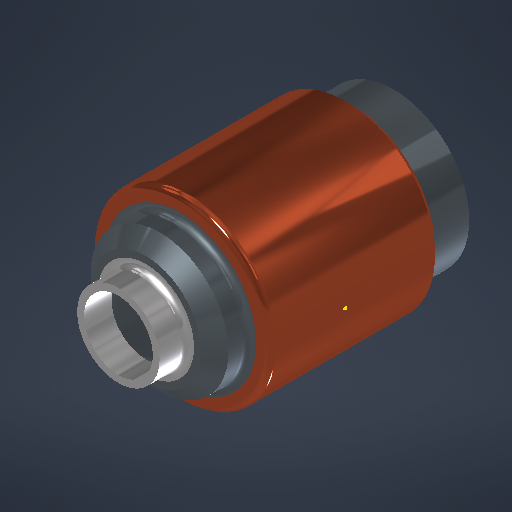
# Autodesk Inventor part: LOWER-NOZZLEv2
Saved by Autodesk Inventor 2025.3 (Build 293356030, 356C)
## iProperties
Created: 2025-08-29
Part Number: LOWER-NOZZLEv2
Material: PC/ABS Plastic
Document SubType Name: Modeling
Designer: lstk1ng
Density: 1.1 g/cm^3
Appearance: Smooth - White
Mass: 704.621 g
Surface Area: 1851.7 cm^2
Volume: 640.564 cm^3
Author: lstk1ng
Autodesk Inventor part; units mm, degrees
ref_plane "XZ Plane" through (0, 0, 0) normal (0, 1, 0) x (-1, 0, 0)
ref_plane "XY Plane" through (0, 0, 0) normal (0, 0, 1) x (1, 0, 0)
sketch "Sketch6" plane through (0, 0, 0) normal (0, 1, 0) x (-1, 0, 0)
  line L0 (0, -100) -> (0, 100)
  line L1 (50, -100) -> (50, -65)
  line L2 (60, -60) -> (60, 0.4584)
  line L3 (55, -65) -> (50, -65)
  line L4 (60, 50) -> (45, 50) construction
  line L5 (25, 80) -> (25, 100)
  line L6 (30, 100) -> (30, 85)
  line L7 (55, 55) -> (60, 55)
  line L8 (65, 50) -> (65, -65)
  line L9 (55, -100) -> (50, -100)
  line L10 (30, 100) -> (25, 100)
  line L11 (45, 50) -> (45, 50)
  line L12 (25, 80) -> (25, 80)
  line L13 (45, 50) -> (25, 80)
  arc A0 (65, 50) -> (60, 55) centre (60, 50) ccw
  arc A1 (50, 60) -> (55, 55) centre (55, 60) ccw
  line L14 (65, -65) -> (60, -70)
  line L15 (60, -60) -> (55, -65)
  line L16 (60, 45) -> (60, 45)
  line L17 (55, 50) -> (55, 50)
  line L18 (35, 80) -> (40, 80)
  line L19 (50, 70) -> (50, 60)
  line L20 (40, 80) -> (50, 70)
  line L21 (54.95, -100) -> (54.95, -70)
  line L22 (60, -70) -> (54.95, -70)
  arc A2 (30, 85) -> (35, 80) centre (35, 85) ccw
  arc A3 (60, 0.4584) -> (45, 50) centre (-29.3125, 0.4584) ccw
  point P0 (0, 0)
  point P1 (0, 0)
  point P2 (60, -65)
  point P3 (30, 80)
  point P4 (65, -70)
  point P5 (25, 50)
  point P6 (50, 80)
  dimension "d88" = 200
  dimension "d89" = 35
  dimension "d90" = 115
  dimension "d91" = 100
  dimension "d92" = 120
  dimension "d95" = 50
  dimension "d96" = 20
  dimension "d97" = 30
  dimension "d99" = 5
  dimension "d100" = 5
  dimension "d101" = 5
  dimension "d102" = 5
  dimension "d103" = 5
  dimension "d107" = 10
  dimension "d108" = 10
  dimension "d109" = 109.9
  dimension "d127" = 5
  constraints: 46 end point, 14 point on line, 8 point on circle, 7 tangent, 5 horizontal, 5 vertical, 4 centre point, 4 perpendicular, 1 coincident, 1 midpoint
  measures "d88" distance of L0.start L0.end
  measures "d89" distance of L1.start L1.end
  measures "d90" distance of L4.start point (60, -65)
  measures "d91" diameter of L1 L0
  measures "d92" diameter of L2 L0
  measures "d95" diameter of L5 L0
  measures "d96" distance of L11.end point (25, 50)
  measures "d97" distance of L12.start point (25, 50)
  measures "d99" distance of L8.end point (65, -70)
  measures "d100" distance of L14.end point (65, -70)
  measures "d101" distance of L2.start point (60, -65)
  measures "d102" distance of L3.start point (60, -65)
  measures "d103" distance of L16.end A0.centre
  measures "d107" distance of L18.end point (50, 80)
  measures "d108" distance of L19.start point (50, 80)
  measures "d109" diameter of L21 L0
  measures "d127" radius of A2
revolve "Revolution5" add sketch "Sketch6" angle 360 about axis through (0, 0, -100) along (0, 0, 1)
ref_plane "Work Plane2" through (65, 0, -7.5) normal (1, 0, 0) x (0, 1, 0)
sketch "Sketch17" plane through (65, 0, -7.5) normal (1, 0, 0) x (0, 1, 0)
  point P0 (0, 7.5)
ref_plane "Work Plane5" through (57.6628, -30, -7.5) normal (0, 0, -1) x (-1, 0, 0)
sketch "Sketch19" plane through (57.6628, -30, -7.5) normal (0, 0, -1) x (-1, 0, 0)
  line L0 (-2.3372, 5) -> (-2.3372, 0)
  line L1 (-2.3372, 30) -> (27.6628, 30) construction
  line L2 (0, 60) -> (-2.3372, 60)
  line L3 (-2.3372, 55) -> (-2.3372, 60)
  line L4 (-2.3372, 0) -> (0, 0)
  circle A0 centre (57.6628, 30) radius 65 projected
  point P0 (57.6628, 30)
  dimension "d92" = 120
  dimension "d159" = 90
  constraints: 10 end point, 3 horizontal, 1 perpendicular
  measures "d159" angle of L0 L1
extrude "Extrusion11" [suppressed]
ref_plane "Work Plane6" through (60, 25, -7.5) normal (1, 0, 0) x (0, 0, -1)
sketch "Sketch20" plane through (60, 25, -7.5) normal (1, 0, 0) x (0, 0, -1)
  line L0 (0, 5) -> (0, -55)
  line L1 (50, 0) -> (50, 5) projected
  line L2 (50, 5) -> (50, -55)
  line L3 (0, 5) -> (50, 5) projected
  line L4 (50, 5) -> (0, 5)
  line L5 (50, -55) -> (0, -55) projected
  line L6 (0, -55) -> (50, -55)
  line L7 (0, 5) -> (0, -55)
  circle A0 centre (25, -25) radius 20
  point P0 (-7.5, -25)
  dimension "d92" = 120
  dimension "d170" = 40
  constraints: 10 end point, 4 collinear, 1 centre point
  measures "d170" diameter of A0
extrude "Extrusion12" [suppressed]
sketch "Sketch23" plane through (65, 25, -7.5) normal (1, 0, 0) x (0, 0, -1)
  arc A0 (45, -25) -> (5, -25) centre (25, -25) ccw projected
  circle A1 centre (25, -25) radius 22.5
  arc A2 (5, -25) -> (45, -25) centre (25, -25) ccw projected
  point P0 (-7.5, -25)
  dimension "d171" = 45
  constraints: 1 centre point, 1 coincident
  measures "d171" diameter of A1
extrude "Extrusion14" [suppressed]
sketch "Sketch24" plane through (80, 0, -32.5) normal (1, 0, 0) x (0, 0, -1)
  circle A0 centre (0, 0) radius 20 projected
  circle A1 centre (0, 0) radius 20
  point P0 (-32.5, 0)
  dimension "d174" = 40
  constraints: 1 centre point, 1 coincident
  measures "d174" diameter of A1
extrude "Extrusion15" [suppressed]
fillet "Fillet3" [suppressed]
body "Solid6"
